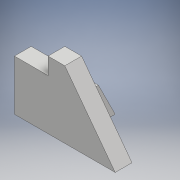
# Autodesk Inventor part: 43
Saved by Autodesk Inventor 2017 (Build 210142000, 142)
## iProperties
Part Number: 43
Material: 一般
Document SubType Name: Modeling
Designer: Brian
Density: 1 g/cm^3
Appearance: 預設
Author: Brian
Autodesk Inventor part; units mm, degrees
ref_plane "YZ Plane" through (0, 0, 0) normal (1, 0, 0) x (0, 1, 0)
ref_plane "XZ Plane" through (0, 0, 0) normal (0, 1, 0) x (-1, 0, 0)
ref_plane "XY Plane" through (0, 0, 0) normal (0, 0, 1) x (1, 0, 0)
sketch "草圖1" plane through (0, 0, 0) normal (0, 1, 0) x (-1, 0, 0)
  line L0 (0, 0) -> (-20, 0)
  line L1 (-20, 0) -> (-20, -30)
  line L2 (-20, -30) -> (0, -30)
  line L3 (0, -30) -> (0, 0)
  line L4 (-20, -30) -> (-60, -30)
  line L5 (-60, -30) -> (-60, 10)
  line L6 (-60, 10) -> (-20, 10)
  line L7 (-20, 10) -> (-20, -30)
  dimension "d0" = 20
  dimension "d1" = 40
  dimension "d2" = 40
  dimension "d3" = 30
  constraints: 16 end point, 4 parallel, 2 horizontal, 2 perpendicular
  measures "d0" distance of L0.start L0.end
  measures "d1" distance of L5.end L6.end
  measures "d2" distance of L6.end L1.end
  measures "d3" distance of L2.end L0.start
extrude "擠出1" add sketch "草圖1" along normal blind 10
chamfer "倒角1" distance 30 distance2 40 1 edges at (60, 5, 10) measured on face at (33.3333, 3.3333, 10)
sketch "草圖2" plane through (0, 0, -30) normal (-1, 0, 0) x (0, 0, 1)
  line L0 (0, 0) -> (0, 10) projected
  line L1 (0, 10) -> (20, 10)
  line L2 (20, 10) -> (20, 30)
  line L3 (20, 30) -> (0, 30)
  line L4 (0, 30) -> (0, 10)
  point P0 (30, 0)
  dimension "d9" = 20
  dimension "d10" = 20
  constraints: 8 end point, 2 parallel, 1 horizontal, 1 perpendicular
  measures "d9" distance of L1.end L2.end
  measures "d10" distance of L2.end L3.end
extrude "擠出2" add sketch "草圖2" against normal blind 30
chamfer "倒角2" distance 20 distance2 10 1 edges at (15, 30, -10) measured on face at (10, 30, -16.6667)
